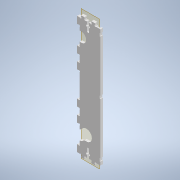
# Autodesk Inventor part: side_top
Saved by Autodesk Inventor 2020 (Build 240168000, 168)
## iProperties
Created: 2020-01-09
Part Number: side_top
Material: Generic
Document SubType Name: Modeling
Designer: erwin
Density: 1 g/cm^3
Appearance: Default
Author: erwin
Autodesk Inventor part; units mm, degrees
ref_plane "YZ Plane" through (0, 0, 0) normal (1, 0, 0) x (0, 1, 0)
ref_plane "XZ Plane" through (0, 0, 0) normal (0, 1, 0) x (-1, 0, 0)
ref_plane "XY Plane" through (0, 0, 0) normal (0, 0, 1) x (1, 0, 0)
ref_plane "Work Plane1" through (0, 0, 0) normal (0, 0, 1) x (1, 0, 0)
sketch "Sketch1" plane through (0, 0, 0) normal (0, 0, 1) x (1, 0, 0)
  line L0 (30, 0) -> (23.9528, 0) projected
  line L1 (30, 0) -> (30, -5) projected
  line L2 (23.9799, -170) -> (30, -170) projected
  line L3 (22, -171.9799) -> (22, -173.6) projected
  line L4 (22, -173.6) -> (17, -173.6) projected
  line L5 (17, -173.6) -> (17, -171.9799) projected
  line L6 (15.0201, -170) -> (13.5, -170) projected
  line L7 (13.5, -170) -> (13.5, -166) projected
  line L8 (13.5, -166) -> (15, -166) projected
  line L9 (15, -166) -> (15, -163.7) projected
  line L10 (15, -163.7) -> (13.5, -163.7) projected
  line L11 (13.5, -163.7) -> (13.5, -157) projected
  line L12 (13.5, -157) -> (10.5, -157) projected
  line L13 (10.5, -157) -> (10.5, -163.7) projected
  line L14 (10.5, -163.7) -> (9, -163.7) projected
  line L15 (9, -163.7) -> (9, -166) projected
  line L16 (9, -166) -> (10.5, -166) projected
  line L17 (10.5, -166) -> (10.5, -170) projected
  line L18 (10.5, -170) -> (8.9799, -170) projected
  line L19 (7, -171.9799) -> (7, -173.6) projected
  line L20 (7, -173.6) -> (2, -173.6) projected
  line L21 (2, -173.6) -> (2, -171.9799) projected
  line L22 (0.0201, -170) -> (-3.6, -170) projected
  line L23 (-3.6, -170) -> (-3.6, -160) projected
  line L24 (-3.6, -160) -> (-1.9799, -160) projected
  line L25 (0, -34.8201) -> (0, -11.9528) projected
  line L26 (-1.9528, -133.2) -> (-3.6, -133.2) projected
  line L27 (-3.6, -133.2) -> (-3.6, -123.2) projected
  line L28 (-3.6, -123.2) -> (-1.9799, -123.2) projected
  line L29 (0, -54.8201) -> (0, -48.7799) projected
  line L30 (-1.9799, -113.2) -> (-3.6, -113.2) projected
  line L31 (-3.6, -113.2) -> (-3.6, -103.2) projected
  line L32 (-3.6, -103.2) -> (-1.9799, -103.2) projected
  line L33 (0, -101.2201) -> (0, -68.7528) projected
  line L34 (-1.9528, -66.8) -> (-3.6, -66.8) projected
  line L35 (-3.6, -66.8) -> (-3.6, -56.8) projected
  line L36 (-3.6, -56.8) -> (-1.9799, -56.8) projected
  line L37 (0, -121.2201) -> (0, -115.1799) projected
  line L38 (-1.9799, -46.8) -> (-3.6, -46.8) projected
  line L39 (-3.6, -46.8) -> (-3.6, -36.8) projected
  line L40 (-3.6, -36.8) -> (-1.9799, -36.8) projected
  line L41 (0, -158.0201) -> (0, -135.1528) projected
  line L42 (-1.9528, -10) -> (-3.6, -10) projected
  line L43 (-3.6, -10) -> (-3.6, 0) projected
  line L44 (-3.6, 0) -> (0.0472, 0) projected
  line L45 (2, 1.9528) -> (2, 3.6) projected
  line L46 (2, 3.6) -> (7, 3.6) projected
  line L47 (7, 3.6) -> (7, 1.9799) projected
  line L48 (8.9799, 0) -> (10.5, 0) projected
  line L49 (10.5, 0) -> (10.5, -4) projected
  line L50 (10.5, -4) -> (9, -4) projected
  line L51 (9, -4) -> (9, -6.3) projected
  line L52 (9, -6.3) -> (10.5, -6.3) projected
  line L53 (10.5, -6.3) -> (10.5, -13) projected
  line L54 (10.5, -13) -> (13.5, -13) projected
  line L55 (13.5, -13) -> (13.5, -6.3) projected
  line L56 (13.5, -6.3) -> (15, -6.3) projected
  line L57 (15, -6.3) -> (15, -4) projected
  line L58 (15, -4) -> (13.5, -4) projected
  line L59 (13.5, -4) -> (13.5, 0) projected
  line L60 (13.5, 0) -> (15.0472, 0) projected
  line L61 (17, 1.9528) -> (17, 3.6) projected
  line L62 (17, 3.6) -> (22, 3.6) projected
  line L63 (22, 3.6) -> (22, 1.9528) projected
  line L64 (29, -165) -> (30, -165) projected
  line L65 (30, -5) -> (29, -5) projected
  line L66 (29, -5) -> (29, -9) projected
  line L67 (29, -9) -> (30, -9) projected
  line L68 (30, -9) -> (30, -83) projected
  line L69 (30, -83) -> (29, -83) projected
  line L70 (29, -83) -> (29, -87) projected
  line L71 (29, -87) -> (30, -87) projected
  line L72 (30, -87) -> (30, -161) projected
  line L73 (30, -161) -> (29, -161) projected
  line L74 (29, -161) -> (29, -165) projected
  arc A0 (17, -171.9799) -> (15.0201, -170) centre (16.0101, -170.9899) ccw projected
  arc A1 (8.9799, -170) -> (7, -171.9799) centre (7.9899, -170.9899) ccw projected
  arc A2 (2, -171.9799) -> (0.0201, -170) centre (1.0101, -170.9899) ccw projected
  arc A3 (-1.9799, -160) -> (0, -158.0201) centre (-0.9899, -159.0101) ccw projected
  arc A4 (0, -135.1528) -> (-1.9528, -133.2) centre (-0.8132, -134.0132) ccw projected
  arc A5 (-1.9799, -123.2) -> (0, -121.2201) centre (-0.9899, -122.2101) ccw projected
  arc A6 (0, -115.1799) -> (-1.9799, -113.2) centre (-0.9899, -114.1899) ccw projected
  arc A7 (-1.9799, -103.2) -> (0, -101.2201) centre (-0.9899, -102.2101) ccw projected
  arc A8 (0, -68.7528) -> (-1.9528, -66.8) centre (-0.8132, -67.6132) ccw projected
  arc A9 (-1.9799, -56.8) -> (0, -54.8201) centre (-0.9899, -55.8101) ccw projected
  arc A10 (0, -48.7799) -> (-1.9799, -46.8) centre (-0.9899, -47.7899) ccw projected
  arc A11 (-1.9799, -36.8) -> (0, -34.8201) centre (-0.9899, -35.8101) ccw projected
  arc A12 (0, -11.9528) -> (-1.9528, -10) centre (-0.8132, -10.8132) ccw projected
  arc A13 (0.0472, 0) -> (2, 1.9528) centre (1.1868, 0.8132) ccw projected
  arc A14 (7, 1.9799) -> (8.9799, 0) centre (7.9899, 0.9899) ccw projected
  arc A15 (15.0472, 0) -> (17, 1.9528) centre (16.1868, 0.8132) ccw projected
  arc A16 (22, 1.9528) -> (23.9528, 0) centre (22.8132, 0.8132) ccw projected
  line L75 (30, -165) -> (30, -170) projected
  arc A17 (23.9799, -170) -> (22, -171.9799) centre (22.9899, -170.9899) ccw projected
  point P0 (0, 0)
  point P1 (22, 0)
  point P2 (22, -170)
  point P3 (17, -170)
  point P4 (7, -170)
  point P5 (2, -170)
  point P6 (0, -160)
  point P7 (0, -133.2)
  point P8 (0, -123.2)
  point P9 (0, -113.2)
  point P10 (0, -103.2)
  point P11 (0, -66.8)
  point P12 (0, -56.8)
  point P13 (0, -46.8)
  point P14 (0, -36.8)
  point P15 (0, -10)
  point P16 (2, 0)
  point P17 (7, 0)
  point P18 (17, 0)
  constraints: 6 other
extrude "Extrusion1" add sketch "Sketch1" along normal blind 3.6
sketch "Sketch3" plane through (0, 0, 0) normal (0, 0, -1) x (-1, 0, 0)
  line L0 (-28, -170) -> (-24, -170) projected
  line L1 (-28, 0) -> (-28, -170) projected
  line L2 (-24, 0) -> (-28, 0) projected
  line L3 (-24, 0) -> (-24, -170) projected
  point P0 (0, 0)
extrude "Extrusion3" cut sketch "Sketch3" against normal blind 1.8
sketch "Sketch16" plane through (0, 0, 3.6) normal (0, 0, 1) x (1, 0, 0)
  line L0 (30, -87) -> (29, -87) projected
  line L1 (29, -87) -> (29, -83) projected
  line L2 (29, -83) -> (30, -83) projected
  line L3 (30, -83) -> (30, -9) projected
  line L4 (30, -9) -> (29, -9) projected
  line L5 (29, -9) -> (29, -5) projected
  line L6 (29, -5) -> (30, -5) projected
  line L7 (30, -5) -> (30, 0) projected
  line L8 (30, 0) -> (23.9528, 0) projected
  arc A0 (22, 1.9528) -> (23.9528, 0) centre (22.8132, 0.8132) ccw projected
  line L9 (22, 1.9528) -> (22, 3.6) projected
  line L10 (22, 3.6) -> (17, 3.6) projected
  line L11 (17, 3.6) -> (17, 1.9528) projected
  arc A1 (15.0472, 0) -> (17, 1.9528) centre (16.1868, 0.8132) ccw projected
  line L12 (15.0472, 0) -> (13.5, 0) projected
  line L13 (13.5, 0) -> (13.5, -4) projected
  line L14 (13.5, -4) -> (15, -4) projected
  line L15 (15, -4) -> (15, -6.3) projected
  line L16 (15, -6.3) -> (13.5, -6.3) projected
  line L17 (13.5, -6.3) -> (13.5, -13) projected
  line L18 (13.5, -13) -> (10.5, -13) projected
  line L19 (10.5, -13) -> (10.5, -6.3) projected
  line L20 (10.5, -6.3) -> (9, -6.3) projected
  line L21 (9, -6.3) -> (9, -4) projected
  line L22 (9, -4) -> (10.5, -4) projected
  line L23 (10.5, -4) -> (10.5, 0) projected
  line L24 (10.5, 0) -> (8.9799, 0) projected
  arc A2 (7, 1.9799) -> (8.9799, 0) centre (7.9899, 0.9899) ccw projected
  line L25 (7, 1.9799) -> (7, 3.6) projected
  line L26 (7, 3.6) -> (2, 3.6) projected
  line L27 (2, 3.6) -> (2, 1.9528) projected
  arc A3 (0.0472, 0) -> (2, 1.9528) centre (1.1868, 0.8132) ccw projected
  line L28 (0.0472, 0) -> (-3.6, 0) projected
  line L29 (-3.6, 0) -> (-3.6, -10) projected
  line L30 (-3.6, -10) -> (-1.9528, -10) projected
  arc A4 (0, -11.9528) -> (-1.9528, -10) centre (-0.8132, -10.8132) ccw projected
  line L31 (0, -11.9528) -> (0, -34.8201) projected
  arc A5 (-1.9799, -36.8) -> (0, -34.8201) centre (-0.9899, -35.8101) ccw projected
  line L32 (-1.9799, -36.8) -> (-3.6, -36.8) projected
  line L33 (-3.6, -36.8) -> (-3.6, -46.8) projected
  line L34 (-3.6, -46.8) -> (-1.9799, -46.8) projected
  arc A6 (0, -48.7799) -> (-1.9799, -46.8) centre (-0.9899, -47.7899) ccw projected
  line L35 (0, -48.7799) -> (0, -54.8201) projected
  arc A7 (-1.9799, -56.8) -> (0, -54.8201) centre (-0.9899, -55.8101) ccw projected
  line L36 (-1.9799, -56.8) -> (-3.6, -56.8) projected
  line L37 (-3.6, -56.8) -> (-3.6, -66.8) projected
  line L38 (-3.6, -66.8) -> (-1.9528, -66.8) projected
  arc A8 (0, -68.7528) -> (-1.9528, -66.8) centre (-0.8132, -67.6132) ccw projected
  line L39 (0, -68.7528) -> (0, -101.2201) projected
  arc A9 (-1.9799, -103.2) -> (0, -101.2201) centre (-0.9899, -102.2101) ccw projected
  line L40 (-1.9799, -103.2) -> (-3.6, -103.2) projected
  line L41 (-3.6, -103.2) -> (-3.6, -113.2) projected
  line L42 (-3.6, -113.2) -> (-1.9799, -113.2) projected
  arc A10 (0, -115.1799) -> (-1.9799, -113.2) centre (-0.9899, -114.1899) ccw projected
  line L43 (0, -115.1799) -> (0, -121.2201) projected
  arc A11 (-1.9799, -123.2) -> (0, -121.2201) centre (-0.9899, -122.2101) ccw projected
  line L44 (-1.9799, -123.2) -> (-3.6, -123.2) projected
  line L45 (-3.6, -123.2) -> (-3.6, -133.2) projected
  line L46 (-3.6, -133.2) -> (-1.9528, -133.2) projected
  arc A12 (0, -135.1528) -> (-1.9528, -133.2) centre (-0.8132, -134.0132) ccw projected
  line L47 (0, -135.1528) -> (0, -158.0201) projected
  arc A13 (-1.9799, -160) -> (0, -158.0201) centre (-0.9899, -159.0101) ccw projected
  line L48 (-1.9799, -160) -> (-3.6, -160) projected
  line L49 (-3.6, -160) -> (-3.6, -170) projected
  line L50 (-3.6, -170) -> (0.0201, -170) projected
  arc A14 (2, -171.9799) -> (0.0201, -170) centre (1.0101, -170.9899) ccw projected
  line L51 (2, -171.9799) -> (2, -173.6) projected
  line L52 (2, -173.6) -> (7, -173.6) projected
  line L53 (7, -173.6) -> (7, -171.9799) projected
  arc A15 (8.9799, -170) -> (7, -171.9799) centre (7.9899, -170.9899) ccw projected
  line L54 (8.9799, -170) -> (10.5, -170) projected
  line L55 (10.5, -170) -> (10.5, -166) projected
  line L56 (10.5, -166) -> (9, -166) projected
  line L57 (9, -166) -> (9, -163.7) projected
  line L58 (9, -163.7) -> (10.5, -163.7) projected
  line L59 (10.5, -163.7) -> (10.5, -157) projected
  line L60 (10.5, -157) -> (13.5, -157) projected
  line L61 (13.5, -157) -> (13.5, -163.7) projected
  line L62 (13.5, -163.7) -> (15, -163.7) projected
  line L63 (15, -163.7) -> (15, -166) projected
  line L64 (15, -166) -> (13.5, -166) projected
  line L65 (13.5, -166) -> (13.5, -170) projected
  line L66 (13.5, -170) -> (15.0201, -170) projected
  arc A16 (17, -171.9799) -> (15.0201, -170) centre (16.0101, -170.9899) ccw projected
  line L67 (17, -171.9799) -> (17, -173.6) projected
  line L68 (17, -173.6) -> (22, -173.6) projected
  line L69 (22, -173.6) -> (22, -171.9799) projected
  arc A17 (23.9799, -170) -> (22, -171.9799) centre (22.9899, -170.9899) ccw projected
  line L70 (23.9799, -170) -> (30, -170) projected
  line L71 (30, -170) -> (30, -165) projected
  line L72 (30, -165) -> (29, -165) projected
  line L73 (29, -165) -> (29, -161) projected
  line L74 (29, -161) -> (30, -161) projected
  line L75 (30, -161) -> (30, -87) projected
  line L76 (0, -30.4) -> (-3.6, -30.4) projected
  line L77 (0, -16.4) -> (-3.6, -16.4) projected
  line L78 (-3.6, -23.3865) -> (2.4, -23.3865) construction
  line L79 (-3.6, -16.3729) -> (2.4, -16.3729)
  line L80 (2.4, -30.4) -> (-3.6, -30.4)
  arc A18 (-3.6, -16.3729) -> (-3.6, -30.4) centre (-3.6, -23.3865) ccw
  arc A19 (2.4, -30.4) -> (2.4, -16.3729) centre (2.4, -23.3865) ccw
  point P0 (0, 0)
  point P1 (-0.6, -23.3865)
  dimension "d39" = 6
  constraints: 8 end point, 4 point on circle, 4 tangent, 2 centre point, 1 midpoint, 1 parallel, 1 perpendicular
  measures "d39" distance of L78.start L78.end
extrude "Extrusion6" cut sketch "Sketch16" against normal through all contours L79 A19 L80 L31 | L31 L76 A18 L79
sketch "Sketch17" plane through (0, 0, 3.6) normal (0, 0, 1) x (1, 0, 0)
  line L0 (0, -16.3729) -> (2.4, -16.3729) projected
  arc A0 (2.4, -30.4) -> (2.4, -16.3729) centre (2.4, -23.3865) ccw projected
  line L1 (2.4, -30.4) -> (0, -30.4) projected
  line L2 (0, -30.4) -> (0, -34.8201) projected
  arc A1 (-1.9799, -36.8) -> (0, -34.8201) centre (-0.9899, -35.8101) ccw projected
  line L3 (-1.9799, -36.8) -> (-3.6, -36.8) projected
  line L4 (-3.6, -36.8) -> (-3.6, -46.8) projected
  line L5 (-3.6, -46.8) -> (-1.9799, -46.8) projected
  arc A2 (0, -48.7799) -> (-1.9799, -46.8) centre (-0.9899, -47.7899) ccw projected
  line L6 (0, -48.7799) -> (0, -54.8201) projected
  arc A3 (-1.9799, -56.8) -> (0, -54.8201) centre (-0.9899, -55.8101) ccw projected
  line L7 (-1.9799, -56.8) -> (-3.6, -56.8) projected
  line L8 (-3.6, -56.8) -> (-3.6, -66.8) projected
  line L9 (-3.6, -66.8) -> (-1.9528, -66.8) projected
  arc A4 (0, -68.7528) -> (-1.9528, -66.8) centre (-0.8132, -67.6132) ccw projected
  line L10 (0, -68.7528) -> (0, -101.2201) projected
  arc A5 (-1.9799, -103.2) -> (0, -101.2201) centre (-0.9899, -102.2101) ccw projected
  line L11 (-1.9799, -103.2) -> (-3.6, -103.2) projected
  line L12 (-3.6, -103.2) -> (-3.6, -113.2) projected
  line L13 (-3.6, -113.2) -> (-1.9799, -113.2) projected
  arc A6 (0, -115.1799) -> (-1.9799, -113.2) centre (-0.9899, -114.1899) ccw projected
  line L14 (0, -115.1799) -> (0, -121.2201) projected
  arc A7 (-1.9799, -123.2) -> (0, -121.2201) centre (-0.9899, -122.2101) ccw projected
  line L15 (-1.9799, -123.2) -> (-3.6, -123.2) projected
  line L16 (-3.6, -123.2) -> (-3.6, -133.2) projected
  line L17 (-3.6, -133.2) -> (-1.9528, -133.2) projected
  arc A8 (0, -135.1528) -> (-1.9528, -133.2) centre (-0.8132, -134.0132) ccw projected
  line L18 (0, -135.1528) -> (0, -158.0201) projected
  arc A9 (-1.9799, -160) -> (0, -158.0201) centre (-0.9899, -159.0101) ccw projected
  line L19 (-1.9799, -160) -> (-3.6, -160) projected
  line L20 (-3.6, -160) -> (-3.6, -170) projected
  line L21 (-3.6, -170) -> (0.0201, -170) projected
  arc A10 (2, -171.9799) -> (0.0201, -170) centre (1.0101, -170.9899) ccw projected
  line L22 (2, -171.9799) -> (2, -173.6) projected
  line L23 (2, -173.6) -> (7, -173.6) projected
  line L24 (7, -173.6) -> (7, -171.9799) projected
  arc A11 (8.9799, -170) -> (7, -171.9799) centre (7.9899, -170.9899) ccw projected
  line L25 (8.9799, -170) -> (10.5, -170) projected
  line L26 (10.5, -170) -> (10.5, -166) projected
  line L27 (10.5, -166) -> (9, -166) projected
  line L28 (9, -166) -> (9, -163.7) projected
  line L29 (9, -163.7) -> (10.5, -163.7) projected
  line L30 (10.5, -163.7) -> (10.5, -157) projected
  line L31 (10.5, -157) -> (13.5, -157) projected
  line L32 (13.5, -157) -> (13.5, -163.7) projected
  line L33 (13.5, -163.7) -> (15, -163.7) projected
  line L34 (15, -163.7) -> (15, -166) projected
  line L35 (15, -166) -> (13.5, -166) projected
  line L36 (13.5, -166) -> (13.5, -170) projected
  line L37 (13.5, -170) -> (15.0201, -170) projected
  arc A12 (17, -171.9799) -> (15.0201, -170) centre (16.0101, -170.9899) ccw projected
  line L38 (17, -171.9799) -> (17, -173.6) projected
  line L39 (17, -173.6) -> (22, -173.6) projected
  line L40 (22, -173.6) -> (22, -171.9799) projected
  arc A13 (23.9799, -170) -> (22, -171.9799) centre (22.9899, -170.9899) ccw projected
  line L41 (23.9799, -170) -> (30, -170) projected
  line L42 (30, -170) -> (30, -165) projected
  line L43 (30, -165) -> (29, -165) projected
  line L44 (29, -165) -> (29, -161) projected
  line L45 (29, -161) -> (30, -161) projected
  line L46 (30, -161) -> (30, -87) projected
  line L47 (30, -87) -> (29, -87) projected
  line L48 (29, -87) -> (29, -83) projected
  line L49 (29, -83) -> (30, -83) projected
  line L50 (30, -83) -> (30, -9) projected
  line L51 (30, -9) -> (29, -9) projected
  line L52 (29, -9) -> (29, -5) projected
  line L53 (29, -5) -> (30, -5) projected
  line L54 (30, -5) -> (30, 0) projected
  line L55 (30, 0) -> (23.9528, 0) projected
  arc A14 (22, 1.9528) -> (23.9528, 0) centre (22.8132, 0.8132) ccw projected
  line L56 (22, 1.9528) -> (22, 3.6) projected
  line L57 (22, 3.6) -> (17, 3.6) projected
  line L58 (17, 3.6) -> (17, 1.9528) projected
  arc A15 (15.0472, 0) -> (17, 1.9528) centre (16.1868, 0.8132) ccw projected
  line L59 (15.0472, 0) -> (13.5, 0) projected
  line L60 (13.5, 0) -> (13.5, -4) projected
  line L61 (13.5, -4) -> (15, -4) projected
  line L62 (15, -4) -> (15, -6.3) projected
  line L63 (15, -6.3) -> (13.5, -6.3) projected
  line L64 (13.5, -6.3) -> (13.5, -13) projected
  line L65 (13.5, -13) -> (10.5, -13) projected
  line L66 (10.5, -13) -> (10.5, -6.3) projected
  line L67 (10.5, -6.3) -> (9, -6.3) projected
  line L68 (9, -6.3) -> (9, -4) projected
  line L69 (9, -4) -> (10.5, -4) projected
  line L70 (10.5, -4) -> (10.5, 0) projected
  line L71 (10.5, 0) -> (8.9799, 0) projected
  arc A16 (7, 1.9799) -> (8.9799, 0) centre (7.9899, 0.9899) ccw projected
  line L72 (7, 1.9799) -> (7, 3.6) projected
  line L73 (7, 3.6) -> (2, 3.6) projected
  line L74 (2, 3.6) -> (2, 1.9528) projected
  arc A17 (0.0472, 0) -> (2, 1.9528) centre (1.1868, 0.8132) ccw projected
  line L75 (0.0472, 0) -> (-3.6, 0) projected
  line L76 (-3.6, 0) -> (-3.6, -10) projected
  line L77 (-3.6, -10) -> (-1.9528, -10) projected
  arc A18 (0, -11.9528) -> (-1.9528, -10) centre (-0.8132, -10.8132) ccw projected
  line L78 (0, -11.9528) -> (0, -16.3729) projected
  line L79 (0, -153.6) -> (-3.6, -153.6) projected
  line L80 (0, -135.1528) -> (0, -158.0201) projected
  arc A19 (-0.2318, -139.5767) -> (5.2144, -151.2768) centre (0, -146.5865) ccw
  arc A20 (8.7055, -149.9855) -> (3.0039, -137.7368) centre (9.7399, -142.0526) ccw
  arc A21 (-0.2318, -139.5767) -> (3.0039, -137.7368) centre (-0.3641, -135.5789) ccw
  arc A22 (8.7055, -149.9855) -> (5.2144, -151.2768) centre (8.1883, -153.9519) ccw
  point P0 (0, 0)
  point P1 (0, -139.5623)
  dimension "d42" = 16
  dimension "d43" = 4
  constraints: 9 point on circle, 4 centre point, 4 tangent, 1 equal radius, 1 midpoint
  measures "d42" diameter of A20
  measures "d43" radius of A21
extrude "Extrusion7" cut sketch "Sketch17" against normal through all contours A21 A20 A22 A19 L18
equation "\"d0\" = wood_thickness"
equation "\"d7\" = deep_for_sliding_cover"
equation "\"wood_thickness\" = 3.6"
equation "\"deep_for_sliding_cover\" = 1.8"
body "Solid1"
